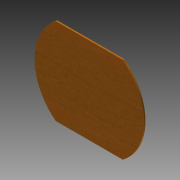
# Autodesk Inventor part: RoofRound
Saved by Autodesk Inventor 2014 SP1 (Build 180222100, 222)
## iProperties
Created: 2015-04-12
Part Number: RoofRound
Material: Wood (Oak)
Document SubType Name: Modeling
Designer: david
Density: 0.76 g/cm^3
Appearance: Yellow Pine - Solid Stained Light Low Gloss
Mass: 399.519 g
Surface Area: 1819.36 cm^2
Volume: 525.683 cm^3
Author: david
Autodesk Inventor part; units mm, degrees
ref_plane "YZ Plane" through (0, 0, 0) normal (1, 0, 0) x (0, 1, 0)
ref_plane "XZ Plane" through (0, 0, 0) normal (0, 1, 0) x (-1, 0, 0)
ref_plane "XY Plane" through (0, 0, 0) normal (0, 0, 1) x (1, 0, 0)
sketch "Sketch1" plane through (0, 0, 0) normal (0, 1, 0) x (-1, 0, 0)
  line L0 (-116.619, 150) -> (116.619, 150)
  line L1 (116.619, -150) -> (-116.619, -150)
  arc A0 (-116.619, 150) -> (-116.619, -150) centre (0, 0) ccw
  arc A1 (116.619, -150) -> (116.619, 150) centre (0, 0) ccw
  dimension "d1" = 300
  dimension "d2" = 190
  dimension "d3" = 190
  constraints: 4 end point, 4 point on circle, 2 centre point, 2 parallel, 1 coincident, 1 horizontal
  measures "d1" distance between parallel lines of L1 L0
  measures "d2" radius of A0
  measures "d3" radius of A1
extrude "Extrusion1" add sketch "Sketch1" along normal blind 5
equation "\"d1\" = Chassis_Body_Length"
equation "\"d2\" = 0.5 * Chassis_Body_Diameter"
equation "\"d3\" = 0.5 * Chassis_Body_Diameter"
equation "\"Chassis_Body_Length\" = 300"
equation "\"Chassis_Body_Diameter\" = 380"
body "Solid1"
